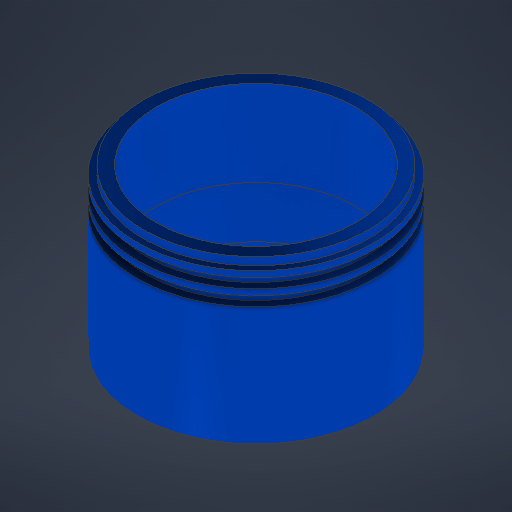
# Autodesk Inventor part: PARTE_EXTERIOR_TOBERA
Saved by Autodesk Inventor 2025 (Build 290162010, 162A)
## iProperties
Created: 2024-07-24
Part Number: PARTE_EXTERIOR_TOBERA
Material: Genérico
Document SubType Name: Modeling
Designer: hansm
Density: 1 g/cm^3
Appearance: Valor por defecto
Author: hansm
Autodesk Inventor part; units mm, degrees
ref_plane "YZ Plane" through (0, 0, 0) normal (1, 0, 0) x (0, 1, 0)
ref_plane "XZ Plane" through (0, 0, 0) normal (0, 1, 0) x (-1, 0, 0)
ref_plane "XY Plane" through (0, 0, 0) normal (0, 0, 1) x (1, 0, 0)
sketch "Boceto1" plane through (0, 0, 0) normal (0, 0, 1) x (1, 0, 0)
  line L0 (-38, 0) -> (-30, 0)
  line L1 (-36, 50.5) -> (-32, 50.5)
  line L2 (-32, 50.5) -> (-32, 23)
  line L3 (-32, 23) -> (-30, 8)
  line L4 (-30, 8) -> (-30, 0)
  line L5 (-36, 50.5) -> (-36, 48)
  line L6 (-36, 48) -> (-38, 48)
  line L7 (-38, 48) -> (-38, 46)
  line L8 (-38, 46) -> (-35.5, 46)
  line L9 (-35.5, 46) -> (-35.5, 43)
  line L10 (-35.5, 43) -> (-38, 43)
  line L11 (-38, 43) -> (-38, 41)
  line L12 (-38, 41) -> (-35.5, 41)
  line L13 (-35.5, 41) -> (-35.5, 38)
  line L14 (-35.5, 38) -> (-38, 38)
  line L15 (-38, 38) -> (-38, 0)
  line L16 (0, -10.1) -> (0, 60.6) projected
  point P0 (0, 0)
  dimension "d1" = 8
  dimension "d2" = 38
  dimension "d3" = 2
  dimension "d4" = 8
  dimension "d5" = 15
  dimension "d6" = 4
  dimension "d26" = 2
  dimension "d27" = 2
  dimension "d28" = 2.5
  dimension "d29" = 2.5
  dimension "d30" = 3
  dimension "d31" = 2
  dimension "d32" = 3
  dimension "d34" = 15
  constraints: 32 end point, 7 perpendicular, 5 point on line, 2 vertical, 1 horizontal, 1 parallel
  measures "d1" distance of L0.start L0.end
  measures "d2" distance of point (0, 0) L0.start
  measures "d3" horizontal distance of L0.end L2.end
  measures "d4" distance of L3.end L0.end
  measures "d5" vertical distance of L3.end L2.end
  measures "d6" distance of L1.start L1.end
  measures "d26" distance of L6.end L7.end
  measures "d27" distance of L5.end L6.end
  measures "d28" distance of L7.end L8.end
  measures "d29" distance of L1.start L5.end
  measures "d30" distance of L8.end L9.end
  measures "d31" distance of L10.end L11.end
  measures "d32" distance of L12.end L13.end
  measures "d34" vertical distance of L14.end L2.end
revolve "Revolución1" add sketch "Boceto1" angle 360 about axis through (0, -10, 0) along (0, 1, 0)
